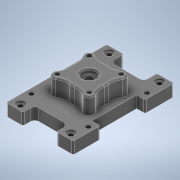
# Autodesk Inventor part: Shoulder base
Saved by Autodesk Inventor 2022 (Build 260153000, 153)
## iProperties
Created: 2022-09-03
Part Number: Shoulder base
Material: Genérico
Document SubType Name: Modeling
Designer: JK
Density: 1 g/cm^3
Appearance: Suave - Negro
Author: JK
Autodesk Inventor part; units mm, degrees
ref_plane "YZ Plane" through (0, 0, 0) normal (1, 0, 0) x (0, 1, 0)
ref_plane "XZ Plane" through (0, 0, 0) normal (0, 1, 0) x (-1, 0, 0)
ref_plane "XY Plane" through (0, 0, 0) normal (0, 0, 1) x (1, 0, 0)
sketch "Boceto1" plane through (0, 0, 0) normal (0, 1, 0) x (-1, 0, 0)
  line L0 (-40, 45) -> (40, 45)
  line L1 (40, 45) -> (40, -45)
  line L2 (40, -45) -> (-40, -45)
  line L3 (-40, -45) -> (-40, 45)
  line L4 (-40, 45) -> (40, -45) construction
  line L5 (40, 45) -> (-40, -45) construction
  circle A0 centre (0, 0) radius 4.35
  dimension "d0" = 80
  dimension "d1" = 90
  dimension "d2" = 8.7
  constraints: 12 end point, 2 midpoint, 2 parallel, 1 centre point, 1 coincident, 1 horizontal, 1 perpendicular
  measures "d0" distance of L1.end L2.end
  measures "d1" distance of L0.end L1.end
  measures "d2" diameter of A0
extrude "Extrusión1" add sketch "Boceto1" along normal blind 14
sketch "Boceto2" plane through (0, 14, 0) normal (0, 1, 0) x (1, 0, 0)
  circle A0 centre (0, 0) radius 4.35 projected
  circle A1 centre (0, 0) radius 8.15
  circle A2 centre (0, 0) radius 4.35 projected
  dimension "d5" = 16.3
  constraints: 1 centre point, 1 coincident, 1 concentric
  measures "d5" diameter of A1
extrude "Extrusión2" [suppressed]
fillet "Empalme1" radius 2 4 edges at (40, 7, -45) (-40, 7, -45) (40, 7, 45) (-40, 7, 45)
sketch "Boceto3" plane through (0, 14, 0) normal (0, 1, 0) x (1, 0, 0)
  circle A0 centre (34, -35) radius 2.7
  circle A1 centre (34, 35) radius 2.7
  circle A2 centre (-34, -35) radius 2.7
  circle A3 centre (-34, 35) radius 2.7
  line L0 (-38, -45) -> (38, -45) projected
  line L1 (40, -43) -> (40, 43) projected
  line L2 (-40, 43) -> (-40, -43) projected
  line L3 (38, 45) -> (-38, 45) projected
  point P0 (0, 0)
  dimension "d9" = 5.4
  dimension "d10" = 10
  dimension "d11" = 6
  dimension "d12" = 6
  dimension "d13" = 10
  constraints: 4 centre point, 3 equal radius, 2 horizontal alignment, 2 vertical alignment
  measures "d9" diameter of A0
  measures "d10" distance from line of L0 A0.centre
  measures "d11" distance from line of L1 A0.centre
  measures "d12" distance from line of L2 A2.centre
  measures "d13" distance from line of A3.centre L3
extrude "Extrusión3" cut sketch "Boceto3" against normal through all
sketch "Boceto4" plane through (0, 0, 0) normal (0, -1, 0) x (1, 0, 0)
  circle A0 centre (34, 35) radius 2.7 projected
  circle A1 centre (34, 35) radius 4.65
  circle A2 centre (-34, 35) radius 2.7 projected
  circle A3 centre (-34, 35) radius 4.65
  circle A4 centre (-34, -35) radius 2.7 projected
  circle A5 centre (-34, -35) radius 4.65
  circle A6 centre (34, -35) radius 2.7 projected
  circle A7 centre (34, -35) radius 4.65
  point P0 (0, 0)
  dimension "d16" = 9.3
  constraints: 4 centre point, 4 coincident, 3 equal radius
  measures "d16" diameter of A1
extrude "Extrusión4" cut sketch "Boceto4" against normal blind 4 contours A0 | A1 | A2 | A3 | A4 | A5 | A6 | A7
sketch "Boceto5" plane through (0, 14, 0) normal (0, 1, 0) x (1, 0, 0)
  circle A0 centre (0, 0) radius 21
  circle A1 centre (0, 0) radius 4.35 projected
  dimension "d19" = 42
  constraints: 1 centre point, 1 coincident
  measures "d19" diameter of A0
extrude "Extrusión5" add sketch "Boceto5" along normal blind 20
sketch "Boceto6" plane through (0, 34, 0) normal (0, 1, 0) x (1, 0, 0)
  circle A0 centre (0, 0) radius 8.125
  dimension "d22" = 16.25
  constraints: 1 centre point, 1 coincident
  measures "d22" diameter of A0
extrude "Extrusión6" cut sketch "Boceto6" against normal blind 5
fillet "Empalme3" radius 2 1 edges at (-8.125, 34, 0)
sketch "Boceto7" plane through (0, 0, 0) normal (0, -1, 0) x (1, 0, 0)
  circle A0 centre (-19, 19) radius 2.7
  circle A1 centre (0, 0) radius 26.87
  line L0 (-26.87, 0) -> (0, 0)
  line L1 (0, 0) -> (-19, 19)
  dimension "d27" = 53.74
  dimension "d28" = 45
  dimension "d29" = 5.4
  constraints: 4 end point, 2 centre point, 2 point on circle, 1 coincident, 1 horizontal
  measures "d27" diameter of A1
  measures "d28" angle of L1 L0
  measures "d29" diameter of A0
extrude "Extrusión7" cut sketch "Boceto7" against normal through all contours A0 L1 A1 | A1 A0 | A0 A1 L1
sketch "Boceto8" plane through (0, 0, 0) normal (0, -1, 0) x (1, 0, 0)
  circle A0 centre (-19, 19) radius 2.7 projected
  line L0 (-14.3812, 19) -> (-16.6906, 15)
  line L1 (-16.6906, 15) -> (-21.3094, 15)
  line L2 (-21.3094, 15) -> (-23.6188, 19)
  line L3 (-23.6188, 19) -> (-21.3094, 23)
  line L4 (-21.3094, 23) -> (-16.6906, 23)
  line L5 (-16.6906, 23) -> (-14.3812, 19)
  circle A1 centre (-19, 19) radius 4
  point P0 (0, 0)
  dimension "d32" = 8
  constraints: 12 end point, 2 coincident, 1 centre point, 1 horizontal alignment, 1 tangent, 13 other
  measures "d32" diameter of A1
extrude "Extrusión8" cut sketch "Boceto8" against normal blind 4 contours A0 | L0 A1 L5 | L0 L1 A1 | A1 | A1 L4 L5 | L1 L2 A1 | A1 L3 L4 | L2 L3 A1
pattern_circular "Patrón circular1" count 4 over 360 about axis through (0, 0, 0) along (0, 1, 0) of "Extrusión7", "Extrusión8"
sketch "Boceto9" plane through (0, 14, 0) normal (0, 1, 0) x (1, 0, 0)
  circle A0 centre (-19, 19) radius 2.7 projected
  circle A1 centre (-19, 19) radius 5.5
  circle A2 centre (0, 0) radius 5.5
  line L0 (-22.889, 15.1109) -> (-3.8891, -3.8891)
  line L1 (-15.1109, 22.889) -> (3.8891, 3.8891)
  circle A3 centre (0, 0) radius 21 projected
  circle A4 centre (0, 0) radius 10.125 projected
  point P0 (-18.22, 10.4418)
  point P1 (-10.4418, 18.22)
  dimension "d38" = 11
  dimension "d44" = 11
  constraints: 4 end point, 4 point on circle, 4 tangent, 2 centre point, 2 coincident
  measures "d38" diameter of A1
  measures "d44" diameter of A2
extrude "Extrusión9" add sketch "Boceto9" along normal up to surface (20 mm away) contours A1 | A1 L1 A3 L0
pattern_circular "Patrón circular2" count 4 over 360 about axis through (0, 14, 0) along (0, 1, 0) of "Extrusión9"
fillet "Empalme4" radius 20 8 edges at (-18.22, 24, -10.4418) (-10.4418, 24, -18.22) (10.4418, 24, -18.22) (18.22, 24, -10.4418) (18.22, 24, 10.4418) (10.4418, 24, 18.22) (-10.4418, 24, 18.22) (-18.22, 24, 10.4418)
fillet "Empalme5" radius 2 16 edges at (9.7004, 34, 21.0773) (22.889, 34, 22.889) (21.0773, 34, 9.7004) (20.9526, 34, -1.4104) (20.9526, 34, 1.4104) (21.0773, 34, -9.7004) (22.889, 34, -22.889) (9.7004, 34, -21.0773) (0, 34, -21) (-9.7004, 34, -21.0773) (-22.889, 34, -22.889) (-21.0773, 34, -9.7004) (-21, 34, 0) (0, 34, 21) (-9.7004, 34, 21.0773) (-22.889, 34, 22.889)
sketch "Boceto10" plane through (0, 4, 0) normal (0, -1, 0) x (1, 0, 0)
  line L0 (-23, -16.6906) -> (-19, -14.3812) projected
  line L1 (-19, -14.3812) -> (-15, -16.6906) projected
  line L2 (-15, -16.6906) -> (-15, -21.3094) projected
  line L3 (-15, -21.3094) -> (-19, -23.6188) projected
  line L4 (-19, -23.6188) -> (-23, -21.3094) projected
  line L5 (-23, -21.3094) -> (-23, -16.6906) projected
  line L6 (16.6906, -23) -> (14.3812, -19) projected
  line L7 (14.3812, -19) -> (16.6906, -15) projected
  line L8 (16.6906, -15) -> (21.3094, -15) projected
  line L9 (21.3094, -15) -> (23.6188, -19) projected
  line L10 (23.6188, -19) -> (21.3094, -23) projected
  line L11 (21.3094, -23) -> (16.6906, -23) projected
  line L12 (23, 16.6906) -> (19, 14.3812) projected
  line L13 (19, 14.3812) -> (15, 16.6906) projected
  line L14 (15, 16.6906) -> (15, 21.3094) projected
  line L15 (15, 21.3094) -> (19, 23.6188) projected
  line L16 (19, 23.6188) -> (23, 21.3094) projected
  line L17 (23, 21.3094) -> (23, 16.6906) projected
  line L18 (-16.6906, 23) -> (-14.3812, 19) projected
  line L19 (-14.3812, 19) -> (-16.6906, 15) projected
  line L20 (-16.6906, 15) -> (-21.3094, 15) projected
  line L21 (-21.3094, 15) -> (-23.6188, 19) projected
  line L22 (-23.6188, 19) -> (-21.3094, 23) projected
  line L23 (-21.3094, 23) -> (-16.6906, 23) projected
  circle A0 centre (-34, -35) radius 4.65 projected
  circle A1 centre (-34, 35) radius 4.65 projected
  circle A2 centre (34, -35) radius 4.65 projected
  circle A3 centre (34, 35) radius 4.65 projected
  arc A4 (-38, 45) -> (-40, 43) centre (-38, 43) ccw projected
  line L24 (-40, -43) -> (-40, 43) projected
  arc A5 (-40, -43) -> (-38, -45) centre (-38, -43) ccw projected
  line L25 (38, -45) -> (-38, -45) projected
  arc A6 (38, -45) -> (40, -43) centre (38, -43) ccw projected
  line L26 (40, 43) -> (40, -43) projected
  arc A7 (40, 43) -> (38, 45) centre (38, 43) ccw projected
  line L27 (-38, 45) -> (38, 45) projected
  circle A8 centre (0, 0) radius 4.35 projected
extrude "Extrusión10" cut sketch "Boceto10" against normal blind 20 contours L0 L1 L2 L3 L4 L5 | L6 L7 L8 L9 L10 L11 | L12 L13 L14 L15 L16 L17 | L18 L19 L20 L21 L22 L23
sketch "Boceto11" plane through (0, 14, 0) normal (0, 1, 0) x (1, 0, 0)
  line L0 (30, -26.67) -> (50, -26.67)
  line L1 (50, -26.67) -> (50, 26.67)
  line L2 (50, 26.67) -> (30, 26.67)
  line L3 (30, 26.67) -> (30, -26.67)
  line L4 (40, -43) -> (40, 43) projected
  line L5 (30, -26.67) -> (50, 26.67) construction
  line L6 (50, -26.67) -> (30, 26.67) construction
  point P0 (0, 0)
  point P1 (40, 0)
  point P2 (40, -26.67)
  point P3 (40, 26.67)
  dimension "d49" = 53.34
  dimension "d50" = 20
  constraints: 12 end point, 3 midpoint, 2 parallel, 1 horizontal, 1 perpendicular
  measures "d49" distance of L0.end L1.end
  measures "d50" distance of L1.end L2.end
extrude "Extrusión11" cut sketch "Boceto11" against normal through all contours L3 L2 L4 L0
fillet "Empalme6" radius 2 2 edges at (40, 7, 26.67) (40, 7, -26.67)
sketch "Boceto12" plane through (0, 0, 0) normal (0, -1, 0) x (1, 0, 0)
  line L0 (40, 43) -> (20, 43)
  line L1 (20, 43) -> (20, 59)
  line L2 (20, 59) -> (40, 59)
  line L3 (40, 59) -> (40, 43)
  arc A0 (-38, 45) -> (-40, 43) centre (-38, 43) ccw projected
  line L4 (-40, 43) -> (-20, 43)
  line L5 (-20, 43) -> (-20, 59)
  line L6 (-20, 59) -> (-40, 59)
  line L7 (-40, 59) -> (-40, 43)
  arc A1 (38, -45) -> (40, -43) centre (38, -43) ccw projected
  line L8 (40, -43) -> (20, -43)
  line L9 (20, -43) -> (20, -60.9524)
  line L10 (20, -60.9524) -> (40, -60.9524)
  line L11 (40, -60.9524) -> (40, -43)
  arc A2 (-40, -43) -> (-38, -45) centre (-38, -43) ccw projected
  line L12 (-40, -43) -> (-20, -43)
  line L13 (-20, -43) -> (-20, -60.9524)
  line L14 (-20, -60.9524) -> (-40, -60.9524)
  line L15 (-40, -60.9524) -> (-40, -43)
  line L16 (-38, 45) -> (38, 45) projected
  point P0 (0, 0)
  point P1 (-20, 45)
  dimension "d54" = 20
  dimension "d55" = 20
  dimension "d56" = 14
  constraints: 32 end point, 8 parallel, 4 collinear, 4 horizontal, 4 perpendicular
  measures "d54" distance of L1.end L2.end
  measures "d55" distance between parallel lines of L7 L5
  measures "d56" distance between parallel lines of L16 L2
extrude "Extrusión12" add sketch "Boceto12" against normal up to surface (14 mm away) contours L0 L1 L2 L3 | A0 L7 L6 L5 L16 | L11 L10 L9 L8 | L12 L13 L14 L15
fillet "Empalme7" radius 2 8 edges at (-40, 7, -60.9524) (-20, 7, -60.9524) (20, 7, -60.9524) (40, 7, -60.9524) (20, 7, 59) (40, 7, 59) (-20, 7, 59) (-40, 7, 59)
fillet "Empalme8" radius 5 4 edges at (-20, 7, 45) (20, 7, 45) (20, 7, -45) (-20, 7, -45)
sketch "Boceto13" plane through (0, 14, 0) normal (0, 1, 0) x (1, 0, 0)
  circle A0 centre (-30, -52) radius 2.7
  circle A1 centre (30, -52) radius 2.7
  circle A2 centre (-30, 53.9524) radius 2.7
  circle A3 centre (30, 53.9524) radius 2.7
  line L0 (-22, -59) -> (-38, -59) projected
  line L1 (40, -57) -> (40, -28.67) projected
  line L2 (-40, -57) -> (-40, 58.9524) projected
  line L3 (-38, 60.9524) -> (-22, 60.9524) projected
  point P0 (0, 0)
  dimension "d61" = 5.4
  dimension "d62" = 7
  dimension "d63" = 10
  dimension "d64" = 10
  dimension "d65" = 7
  constraints: 4 centre point, 3 equal radius, 2 horizontal alignment, 2 vertical alignment
  measures "d61" diameter of A0
  measures "d62" distance from line of A0.centre L0
  measures "d63" distance from line of A1.centre L1
  measures "d64" distance from line of L2 A0.centre
  measures "d65" distance from line of L3 A2.centre
extrude "Extrusión13" cut sketch "Boceto13" against normal through all
sketch "Boceto14" plane through (0, 14, 0) normal (0, 1, 0) x (1, 0, 0)
  circle A0 centre (-30, -52) radius 2.7 projected
  circle A1 centre (-30, -52) radius 5
  circle A2 centre (30, -52) radius 2.7 projected
  circle A3 centre (30, -52) radius 5
  circle A4 centre (-30, 53.9524) radius 2.7 projected
  circle A5 centre (-30, 53.9524) radius 5
  circle A6 centre (30, 53.9524) radius 2.7 projected
  circle A7 centre (30, 53.9524) radius 5
  point P0 (0, 0)
  dimension "d68" = 10
  constraints: 4 centre point, 4 coincident, 3 equal radius
  measures "d68" diameter of A1
extrude "Extrusión14" cut sketch "Boceto14" against normal blind 2 contours A0 | A1 | A2 | A3 | A4 | A5 | A6 | A7
